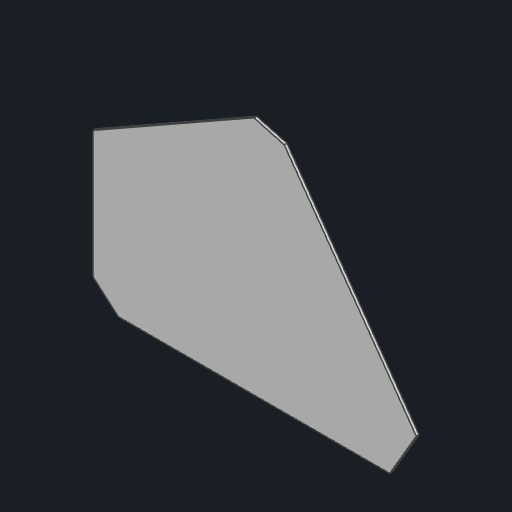
# Autodesk Inventor part: SideChestPanel
Saved by Autodesk Inventor 2025.2 (Build 292293000, 293)
## iProperties
Created: 2025-10-06
Part Number: SideChestPanel
Material: Generic
Document SubType Name: Sheet Metal
Designer: valer
Density: 1 g/cm^3
Sheet Metal Rule: Default
Appearance: Default
Author: valer
Autodesk Inventor part; units mm, degrees
ref_plane "YZ Plane" through (0, 0, 0) normal (1, 0, 0) x (0, 1, 0)
ref_plane "XZ Plane" through (0, 0, 0) normal (0, 1, 0) x (-1, 0, 0)
ref_plane "XY Plane" through (0, 0, 0) normal (0, 0, 1) x (1, 0, 0)
sketch "Sketch1" plane through (0, 0, 0) normal (0, 0, 1) x (1, 0, 0)
  line L0 (-369.2095, 28.577) -> (-369.2095, 169.4392)
  line L1 (-369.2095, 169.4392) -> (-190.2343, 271.0426)
  line L2 (-190.2343, 271.0426) -> (-156.6833, 261.9838)
  line L3 (-156.6833, 261.9838) -> (-9.8327, 54.7186)
  line L4 (-9.8327, 54.7186) -> (-39.3108, 4.1742)
  line L5 (-39.3108, 4.1742) -> (-341.1578, 4.1742)
  line L6 (-341.1578, 4.1742) -> (-369.2095, 28.577)
  point P0 (0, 0)
extrude "Plate1" add sketch "Sketch1" along normal blind 3.048
equation "\"d0\" = Thickness"
equation "\"BendRadius\" = Thickness"
equation "\"BendReliefWidth\" = Thickness"
equation "\"BendReliefDepth\" = 0.5 * Thickness"
equation "\"CornerReliefSize\" = 4 * Thickness"
equation "\"MinimumRemnant\" = 2 * Thickness"
equation "\"TransitionRadius\" = BendRadius"
equation "\"JacobiRadiusSize\" = BendRadius"
equation "\"GapSize\" = Thickness"
equation "\"Thickness\" = 3.048"
body "Solid1"
